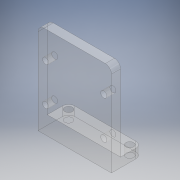
# Autodesk Inventor part: Kamera Holder
Saved by Autodesk Inventor 2017 (Build 210142000, 142)
## iProperties
Created: 2021-02-18
Part Number: Kamera Holder
Material: Generic
Document SubType Name: Modeling
Designer: Lenovo Y900
Density: 1 g/cm^3
Appearance: Polycarbonate - Clear
Author: Lenovo Y900
Autodesk Inventor part; units mm, degrees
ref_plane "YZ Plane" through (0, 0, 0) normal (1, 0, 0) x (0, 1, 0)
ref_plane "XZ Plane" through (0, 0, 0) normal (0, 1, 0) x (-1, 0, 0)
ref_plane "XY Plane" through (0, 0, 0) normal (0, 0, 1) x (1, 0, 0)
sketch "Sketch1" plane through (0, 0, 0) normal (0, 0, 1) x (1, 0, 0)
  line L0 (-12, -5) -> (12, -5)
  line L1 (12, -5) -> (12, 5)
  line L2 (12, 5) -> (-12, 5)
  line L3 (-12, 5) -> (-12, -5)
  line L4 (-12, -5) -> (12, 5) construction
  line L5 (12, -5) -> (-12, 5) construction
  line L6 (-12, 5) -> (-10, 5)
  line L7 (-12, 3) -> (-12, 5)
  line L8 (12, 5) -> (10, 5)
  line L9 (10, 4.25) -> (10, 4.1667)
  line L10 (10, 3) -> (11.25, 3)
  line L11 (12, 3) -> (12, 5)
  circle A0 centre (-10, 3) radius 1.25
  circle A1 centre (10, 3) radius 1.25
  point P0 (0, 0)
  point P1 (-12, 0)
  point P2 (12, 0)
  dimension "d0" = 24
  dimension "d1" = 10
  dimension "d14" = 2.5
  dimension "d15" = 2.5
  dimension "d22" = 20
  constraints: 24 end point, 4 midpoint, 4 parallel, 3 horizontal, 2 centre point, 2 perpendicular, 2 point on circle, 1 coincident, 1 point on line
  measures "d0" distance of L2.end L1.end
  measures "d1" distance of L1.end L0.end
  measures "d14" diameter of A0
  measures "d15" diameter of A1
  measures "d22" distance of L10.start A0.centre
extrude "Extrusion4" add sketch "Sketch1" along normal blind 3
fillet "Fillet1" radius 2 1 edges at (-12, 5, 1.5)
fillet "Fillet2" radius 2 1 edges at (12, 5, 1.5)
sketch "Sketch3" plane through (0, 0, 3) normal (0, 0, 1) x (1, 0, 0)
  line L0 (12, -5) -> (12, 3) projected
  line L1 (12, -5) -> (-12, -5)
  line L2 (-12, -5) -> (-12, -2)
  line L3 (-12, -2) -> (12, -2)
  line L4 (12, -2) -> (12, -5)
  point P0 (0, 0)
  dimension "d24" = 3
  constraints: 8 end point, 2 parallel, 1 horizontal, 1 perpendicular
  measures "d24" distance of L1.end L2.end
extrude "Extrusion5" add sketch "Sketch3" along normal blind 27
sketch "Sketch4" plane through (-12, -2, 3) normal (0, 1, 0) x (1, 0, 0)
  circle A0 centre (21.5, -18.0021) radius 1
  circle A1 centre (2.5, -18.0021) radius 1
  circle A2 centre (21.5, -5.5021) radius 1
  circle A3 centre (2.4716, -5.5021) radius 1
  line L0 (24, -0.0021) -> (0, -0.0021)
  point P0 (12, 3)
  constraints: 4 centre point, 2 end point, 1 horizontal
fillet "Fillet3" radius 2 2 edges at (12, -3.5, 30) (-12, -3.5, 30)
extrude "Extrusion7" cut sketch "Sketch4" against normal blind 3
body "Solid3"
